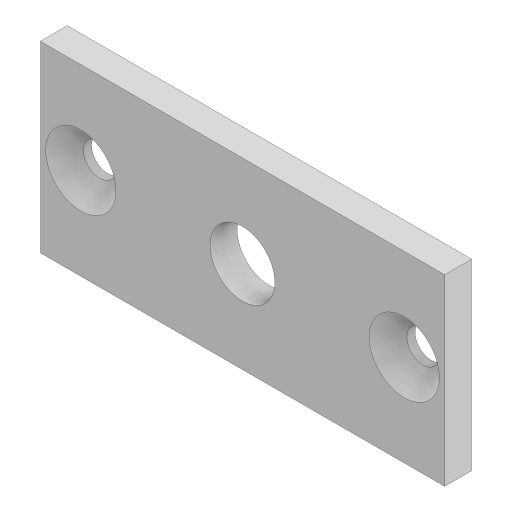
# Autodesk Inventor part: Bearing_mount
Saved by Autodesk Inventor 2023 (Build 270158000, 158)
## iProperties
Created: 2023-10-18
Part Number: Bearing_mount
Material: Generic
Document SubType Name: Modeling
Designer: MVeszpremi
Density: 1 g/cm^3
Appearance: Default
Author: MVeszpremi
Autodesk Inventor part; units mm, degrees
ref_plane "YZ Plane" through (0, 0, 0) normal (1, 0, 0) x (0, 1, 0)
ref_plane "XZ Plane" through (0, 0, 0) normal (0, 1, 0) x (-1, 0, 0)
ref_plane "XY Plane" through (0, 0, 0) normal (0, 0, 1) x (1, 0, 0)
sketch "Sketch1" plane through (0, 0, 0) normal (0, 0, 1) x (1, 0, 0)
  circle A0 centre (0, 0) radius 3
  circle A1 centre (15, 0) radius 1.5
  circle A2 centre (-15, 0) radius 1.5
  line L0 (-18.75, 8.5) -> (18.75, 8.5)
  line L1 (18.75, 8.5) -> (18.75, -8.5)
  line L2 (18.75, -8.5) -> (-18.75, -8.5)
  line L3 (-18.75, -8.5) -> (-18.75, 8.5)
  line L4 (-18.75, 8.5) -> (18.75, -8.5) construction
  line L5 (18.75, 8.5) -> (-18.75, -8.5) construction
  dimension "d0" = 15
  dimension "d1" = 3
  dimension "d2" = 3
  dimension "d3" = 15
  dimension "d4" = 6
  dimension "d5" = 17
  dimension "d6" = 37.5
  constraints: 12 end point, 3 centre point, 2 midpoint, 2 parallel, 1 coincident, 1 horizontal, 1 perpendicular
  measures "d0" distance of A2.centre point (0, 0)
  measures "d1" diameter of A2
  measures "d2" diameter of A1
  measures "d3" distance of A1.centre point (0, 0)
  measures "d4" diameter of A0
  measures "d5" distance between parallel lines of L2 L0
  measures "d6" distance between parallel lines of L1 L3
extrude "Extrusion1" add sketch "Sketch1" along normal blind 2.5
chamfer "Chamfer1" distance 1.75 angle 45 2 edges at (-16.5, 0, 2.5) (13.5, 0, 2.5)
body "Solid1"
